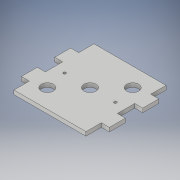
# Autodesk Inventor part: thumper-bumper-top-v2
Saved by Autodesk Inventor 2017 (Build 210142000, 142)
## iProperties
Created: 2017-02-22
Part Number: thumper-bumper-top-v2
Material: Generic
Document SubType Name: Modeling
Designer: John
Density: 1 g/cm^3
Appearance: Default
Author: John
Autodesk Inventor part; units mm, degrees
ref_plane "YZ Plane" through (0, 0, 0) normal (1, 0, 0) x (0, 1, 0)
ref_plane "XZ Plane" through (0, 0, 0) normal (0, 1, 0) x (-1, 0, 0)
ref_plane "XY Plane" through (0, 0, 0) normal (0, 0, 1) x (1, 0, 0)
sketch "Sketch1" plane through (0, 0, 0) normal (0, 1, 0) x (-1, 0, 0)
  line L0 (0, 30) -> (66, 30) construction
  line L1 (66, 36.5) -> (60, 36.5)
  line L2 (60, 36.5) -> (60, 48.5) construction
  line L3 (60, 48.5) -> (66, 48.5)
  line L4 (66, 48.5) -> (66, 36.5)
  line L5 (60, 48.5) -> (60, 60)
  line L6 (60, 60) -> (6, 60)
  line L7 (66, 23.5) -> (60, 23.5)
  line L8 (60, 23.5) -> (60, 11.5) construction
  line L9 (60, 11.5) -> (66, 11.5)
  line L10 (66, 11.5) -> (66, 23.5)
  line L11 (60, 11.5) -> (60, 0)
  line L12 (60, 36.5) -> (60, 23.5)
  line L13 (33, 30) -> (33, 0) construction
  line L14 (0, 36.5) -> (6, 36.5)
  line L15 (6, 36.5) -> (6, 48.5) construction
  line L16 (6, 48.5) -> (0, 48.5)
  line L17 (0, 48.5) -> (0, 36.5)
  line L18 (6, 48.5) -> (6, 60)
  line L19 (0, 23.5) -> (6, 23.5)
  line L20 (6, 23.5) -> (6, 11.5) construction
  line L21 (6, 11.5) -> (0, 11.5)
  line L22 (0, 11.5) -> (0, 23.5)
  line L23 (6, 11.5) -> (6, 0)
  line L24 (6, 36.5) -> (6, 23.5)
  line L25 (6, 0) -> (60, 0)
  dimension "d2" = 6
  dimension "d3" = 12
  dimension "d4" = 18.5
  dimension "d5" = 33
  dimension "d6" = 11.5
  dimension "d7" = 0
  constraints: 52 end point, 15 symmetric about line, 3 parallel, 2 horizontal, 2 midpoint, 2 perpendicular, 2 vertical
  measures "d2" distance of L2.end L3.end
  measures "d3" distance of L1.end L2.end
  measures "d4" distance between parallel lines of L0 L3
  measures "d5" distance between parallel lines of L4 L13
  measures "d6" distance between parallel lines of L6 L3
  measures "d7" distance from line of L0.end L4
extrude "Extrusion1" add sketch "Sketch1" along normal blind 3
sketch "Sketch2" plane through (0, 3, 0) normal (0, 1, 0) x (1, 0, 0)
  line L0 (-6, -36.5) -> (-6, -23.5) projected
  line L1 (-6, -30) -> (-60, -30) construction
  line L2 (-60, -23.5) -> (-60, -36.5) projected
  line L3 (-6, 0) -> (-60, 0) projected
  line L4 (-33, 0) -> (-33, -60) construction
  line L5 (-6, -60) -> (-60, -60) projected
  circle A0 centre (-49, -46) radius 4.5
  circle A1 centre (-17, -14) radius 4.5
  circle A2 centre (-33, -30) radius 4.5
  circle A3 centre (-14, -30) radius 1
  circle A4 centre (-52, -30) radius 1
  point P0 (0, 0)
  dimension "d16" = 9
  dimension "d17" = 9
  dimension "d18" = 16
  dimension "d19" = 16
  dimension "d20" = 16
  dimension "d21" = 16
  dimension "d22" = 9
  dimension "d23" = 2
  dimension "d24" = 2
  dimension "d25" = 19
  dimension "d26" = 19
  constraints: 5 centre point, 5 midpoint, 4 end point, 2 point on line
  measures "d16" diameter of A0
  measures "d17" diameter of A1
  measures "d18" distance from line of L1 A0.centre
  measures "d19" distance from line of L4 A0.centre
  measures "d20" distance from line of L4 A1.centre
  measures "d21" distance from line of L1 A1.centre
  measures "d22" diameter of A2
  measures "d23" diameter of A3
  measures "d24" diameter of A4
  measures "d25" distance of A2.centre A3.centre
  measures "d26" distance of A4.centre A2.centre
extrude "Extrusion2" cut sketch "Sketch2" against normal through all
body "Solid1"
